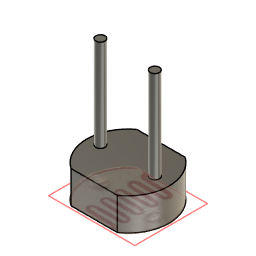
photoresistor v3 (Autodesk Fusion 360 design; units mm, degrees)
Autodesk Fusion 360 part; units mm, degrees
sketch "Sketch2" plane through (0, 0, 0) normal (0, 0, 1) x (1, 0, 0)
  line L0 (-1.5076, -2.2009) -> (1.5076, -2.2009)
  line L1 (-1.5744, 2.1537) -> (1.5744, 2.1537)
  arc A0 (1.5076, -2.2009) -> (1.5744, 2.1537) centre (0, 0) ccw
  arc A1 (-1.5744, 2.1537) -> (-1.5076, -2.2009) centre (0, 0) ccw
  circle A2 centre (-1.9, 0.1) radius 0.3
  circle A3 centre (1.65, 0.1) radius 0.3
  dimension "d3" = 0.6
  dimension "d4" = 0.6
  constraint coincident A0.centre A1.centre
  constraint horizontal L0
  constraint coincident L1.start A0
  constraint parallel L0 L1
  constraint concentric A0 A1
  measures "d3" diameter of A2
  measures "d4" diameter of A3
extrude "Extrude1" add sketch "Sketch2" along normal blind 2.1 contours L0 L1 A0 A1 | A2 | A3
extrude "Extrude2" add sketch "Sketch2" along normal blind 6 from surface at 2.1 contours A2 | A3
